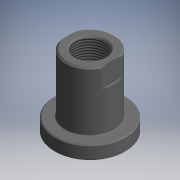
# Autodesk Inventor part: 1559400 EAGF-V2-KF-80/100---(GS)
Saved by Autodesk Inventor 2017.3 (Build 213256000, 256)
## iProperties
Part Number: 1559400 EAGF-V2-KF-80/100---(GS)
Material: Generic
Catalog Web Link: www.cadenas.de
Description: EAGF-V2-KF-(GS)-Gewindestueck
Vendor: FESTO
Document SubType Name: Modeling
Designer: partserver
Manufacturer: FESTO
Mass: 29.0502 g
Surface Area: 93.9672 cm^2
Volume: 29.0502 cm^3
Density: 1 g/cm^3
Appearance: PSOLRGB-128-128-128
Category: PARTsolutions
Company: FESTO
Title: 1559400 EAGF-V2-KF-80/100---(GS)
Author: Cadenas PARTsolutions
Comments: Gewindestueck
PSOL_IDENT_0: {$CADENAS_DATA\23d-libs\festo\parts\e\eagf\parts\eagf_gs.prj},213 {VTYP=3D},{NB=1559400 EAGF-V2-KF-8
PSOL_IDENT_1: 0/100---(GS)},{LINA=1559400 EAGF-V2-KF-80/100---(GS)},{NN=EAGF-V2-KF-(GS)},{DATE=20.07.2020 13:53:58
PSOL_IDENT_2: },{GEOMDATE=17.05.2016 08:04:00},{VERSION=},{LINEID=20},{WBVAR=},{WBNUMERIC=}  {NB=1559400 EAGF-V2-K
PSOL_IDENT_3: F-80/100---(GS)},{LINA=1559400 EAGF-V2-KF-80/100---(GS)},{KT=DUMMY},{TNR=1559400},{TYP=EAGF-V2-KF-80
PSOL_IDENT_4: /100},{D1=44.000},{D2=0.000},{D3=20.000},{D3P=1.500},{D4=30.000},{H1=45.000},{H2=8.450},{H3=12.000},
PSOL_IDENT_5: {T1=30.000},{T2=33.000},{T3=0.000},{R=0.600},{SW=27.000}
NB: 1559400 EAGF-V2-KF-80/100---(GS)
NN: EAGF-V2-KF-(GS)
NT: Gewindestueck
NBSYN: $TNR. $TYP.---(GS)
LINA: 1559400 EAGF-V2-KF-80/100---(GS)
CATALOG: Festo
TNR: 1559400
TYP: EAGF-V2-KF-80/100
D1: 44
D2: 0
D3: 20
D3P: 1.5
D4: 30
H1: 45
H2: 8.45
H3: 12
T1: 30
T2: 33
T3: 0
R: 0.6
SW: 27
SUPPLIER: FESTO
ARTICLENO: 1559400 EAGF-V2-KF-80/100---(GS)
BOMINFO: 1559400 EAGF-V2-KF-80/100---(GS)
CREATOR: CADENAS GmbH
Autodesk Inventor part; units mm, degrees
sketch "Sketch_1" plane through (0, 0, 0) normal (1, 0, 0) x (0, 1, 0)
  line L0 (0, -6.6953) -> (0, 0)
  line L1 (0, 0) -> (21.4, 0)
  line L2 (21.4, 0) -> (22, -0.6)
  line L3 (22, -0.6) -> (22, -7.85)
  line L4 (22, -7.85) -> (21.4, -8.45)
  line L5 (21.4, -8.45) -> (15.6, -8.45)
  arc A0 (15.6, -8.45) -> (15, -9.05) centre (15.6, -9.05) ccw
  line L6 (15, -9.05) -> (15, -44)
  line L7 (15, -44) -> (14, -45)
  line L8 (14, -45) -> (10, -45)
  line L9 (10, -45) -> (9.188, -44.188)
  line L10 (9.188, -44.188) -> (9.188, -12)
  line L11 (9.188, -12) -> (0, -6.6953)
  line L12 (0, -6.6953) -> (0, 0)
  constraints: 26 end point, 2 point on circle, 1 centre point
revolve "Revolution1" add sketch "Sketch_1" angle 360 about axis through (0, 0, -6.6953) along (0, 0, -1)
thread "Thread1" size "M20x1.5" class "6H" standard "ISO Metric profile" length 29.188
sketch "Sketch_4" plane through (0, 0, -45) normal (0, 0, 1) x (1, 0, 0)
  line L0 (-18.5, -27) -> (18.5, -27)
  line L1 (18.5, -27) -> (18.5, 22)
  line L2 (18.5, 22) -> (13.5, 22)
  line L3 (13.5, 22) -> (13.5, -22)
  line L4 (13.5, -22) -> (-13.5, -22)
  line L5 (-13.5, -22) -> (-13.5, 22)
  line L6 (-13.5, 22) -> (-18.5, 22)
  line L7 (-18.5, 22) -> (-18.5, -27)
  constraints: 16 end point
extrude "Extrusion1" cut sketch "Sketch_4" along normal blind 12
ref_plane "ANBAU_XY" through (0, 0, -8.45) normal (0, 0, 1) x (1, 0, 0)
ref_plane "ANBAU_YZ" through (0, 0, -8.45) normal (1, 0, 0) x (0, 1, 0)
ref_plane "ANBAU_ZX" through (0, 0, -8.45) normal (0, 1, 0) x (0, 0, 1)
ref_plane "EP_IP_XY" through (0, 0, 0) normal (0, 0, -1) x (1, 0, 0)
ref_plane "EP_IP_YZ" through (0, 0, 0) normal (1, 0, 0) x (0, -1, 0)
ref_plane "EP_IP_ZX" through (0, 0, 0) normal (0, -1, 0) x (0, 0, -1)
body "Solid1"
